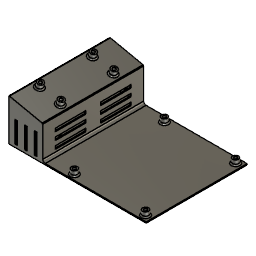
Assembly (Autodesk Fusion 360 archive; units mm, degrees)
design "Chassis"
Autodesk Fusion 360 part; units mm, degrees
sketch "Sketch1" plane through (0, 0, 0) normal (0, 1, 0) x (1, 0, 0)
  line L0 (-55.7763, -66.6431) -> (-54.7763, -66.6431)
  line L1 (-54.7763, -66.6431) -> (0, -55)
  line L2 (0, -55) -> (0, 0)
  line L3 (0, 0) -> (170, 0)
  line L4 (170, 0) -> (170, 2)
  line L5 (170, 2) -> (-55.7763, 2)
  line L6 (-55.7763, 2) -> (-55.7763, -66.6431)
  dimension "d4" = 1
  dimension "d5" = 170
  dimension "d6" = 2
  dimension "d7" = 56
  dimension "d8" = 55
  dimension "d9" = 12
  constraint horizontal L0
  constraint coincident L2.end L3.start
  constraint vertical L2
  constraint perpendicular L2 L3
  constraint perpendicular L3 L4
  constraint perpendicular L4 L5
  constraint perpendicular L0 L6
  measures "d4" distance of L0.start L0.end
  measures "d5" distance of L2.end L3.end
  measures "d6" distance of L3.end L4.end
  measures "d7" distance of L0.end L1.end
  measures "d8" distance of L1.end L2.end
  measures "d9" angle of L1 L3
extrude "Extrude1" add sketch "Sketch1" along normal mid plane 166
fillet "Fillet1" radius 4 1 edges at (0, 0, 0)
chamfer "Chamfer1" distance 1 angle 45 1 edges at (0, 0, 55)
shell "Shell3" thickness 1.8 removed faces 0 bodies 1
sketch "Sketch2" plane through (0, 0, 0) normal (0, 0, 1) x (-1, 0, 0)
  line L0 (-4, -83) -> (-4, 83)
  line L1 (-4, 83) -> (-170, 83)
  line L2 (-170, 83) -> (-170, -83)
  line L3 (-170, -83) -> (-4, -83)
  line L4 (-43, 74) -> (-160, 74) construction
  line L5 (-160, 74) -> (-160, -74) construction
  line L6 (-160, -74) -> (-43, -74) construction
  line L7 (-43, -74) -> (-43, 74) construction
  circle A0 centre (-43, 74) radius 5
  circle A1 centre (-43, -74) radius 5
  circle A2 centre (-160, 74) radius 5
  circle A3 centre (-160, -74) radius 5
  point P0 (-43, 0)
  dimension "d14" = 117
  dimension "d15" = 148
  dimension "d17" = 10
  dimension "d18" = 10
  constraint horizontal L4
  constraint vertical L5
  constraint horizontal L6
  constraint vertical L7
  constraint midpoint L7 P0
  constraint horizontal origin P0
  constraint coincident L4.start L7.end
  constraint coincident L6.end L7.start
  constraint equal A0 A1
  constraint coincident L4.end L5.start
  constraint coincident L5.end L6.start
  constraint equal A0 A2
  constraint equal A0 A3
  measures "d14" distance of L4.start L4.end
  measures "d15" distance of L4.start L6.end
  measures "d17" distance of L2 L5
  measures "d18" diameter of A0
extrude "Extrude2" add sketch "Sketch2" along normal blind 8 contours A0 | A1 | A2 | A3
sketch "Sketch3" plane through (11.1853, 0, 52.6225) normal (0.207912, 0, 0.978148) x (0, 1, 0)
  line L0 (83, 12.4351) -> (83, 67.4351)
  line L1 (83, 67.4351) -> (-83, 67.4351)
  line L2 (-83, 67.4351) -> (-83, 12.4351)
  line L3 (-43.5, 57.4351) -> (43.5, 57.4351) construction
  line L4 (43.5, 57.4351) -> (43.5, 22.4351) construction
  line L5 (43.5, 22.4351) -> (-43.5, 22.4351) construction
  line L6 (-43.5, 22.4351) -> (-43.5, 57.4351) construction
  circle A0 centre (-43.5, 57.4351) radius 5
  circle A1 centre (43.5, 57.4351) radius 5
  circle A2 centre (-43.5, 22.4351) radius 5
  circle A3 centre (43.5, 22.4351) radius 5
  line L7 (-83, 12.4351) -> (83, 12.4351)
  point P0 (0, 22.4351)
  point P1 (0, 10.3528)
  dimension "d21" = 87
  dimension "d22" = 35
  dimension "d23" = 10
  dimension "d24" = 10
  constraint horizontal L3
  constraint vertical L4
  constraint horizontal L5
  constraint vertical L6
  constraint midpoint L5 P0
  constraint vertical P0 P1
  constraint coincident L3.start L6.end
  constraint coincident L3.end L4.start
  constraint coincident L5.end L6.start
  constraint coincident L4.end L5.start
  constraint equal A0 A2
  constraint equal A1 A2
  constraint equal A1 A3
  measures "d21" distance of L3.start L3.end
  measures "d22" distance of L3.start L5.end
  measures "d23" distance of L1 L3
  measures "d24" diameter of A0
extrude "Extrude3" add sketch "Sketch3" along normal blind 8 contours A0 | A1 | A2 | A3
sketch "Sketch5" plane through (12.8486, 0, 60.4477) normal (0.207912, 0, 0.978148) x (0, 1, 0)
  circle A0 centre (-43.5, 57.4351) radius 5
  circle A1 centre (43.5, 57.4351) radius 5
  circle A2 centre (-43.5, 22.4351) radius 5
  circle A3 centre (43.5, 22.4351) radius 5
  point P0 (-43.5, 57.4351)
  point P1 (43.5, 57.4351)
  point P2 (43.5, 22.4351)
  point P3 (-43.5, 22.4351)
  constraint coincident P0 A0.centre
  constraint coincident P1 A1.centre
  constraint coincident P2 A3.centre
  constraint coincident A2.centre P3
hole "Hole1" at (-9.0963, -43.5, 65.1122) at (-43.3315, -43.5, 72.3891) at (-9.0963, 43.5, 65.1122) at (-43.3315, 43.5, 72.3891) direction (-0.207912, 0, -0.978148) diameter 4.5 depth 6 tip angle 180 countersink diameter 5.2 countersink angle 90
sketch "Sketch6" plane through (0, 0, 8) normal (0, 0, 1) x (-1, 0, 0)
  circle A0 centre (-43, 74) radius 5
  circle A1 centre (-43, -74) radius 5
  circle A2 centre (-160, -74) radius 5
  circle A3 centre (-160, 74) radius 5
  point P0 (-43, -74)
  point P1 (-160, -74)
  point P2 (-43, 74)
  point P3 (-160, 74)
  constraint coincident P0 A1.centre
  constraint coincident P1 A2.centre
  constraint coincident P2 A0.centre
  constraint coincident P3 A3.centre
hole "Hole2" at (43, -74, 8) at (43, 74, 8) at (160, 74, 8) at (160, -74, 8) direction (0, 0, -1) diameter 4.5 depth 6 tip angle 180 countersink diameter 5.2 countersink angle 90
fillet "Fillet3" radius 2 4 edges at (47.6616, -75.8081, 0) (47.6616, 72.1919, 0) (164.6616, -75.8081, 0) (164.6616, 72.1919, 0)
fillet "Fillet4" radius 2 4 edges at (-46.7634, 38.8384, 64.9399) (-46.7634, -48.1616, 64.9399) (-12.5282, -48.1616, 57.6629) (-12.5282, 38.8384, 57.6629)
sketch "Sketch8" plane through (-55.7763, 0, 0) normal (-1, 0, 0) x (0, -1, 0)
  line L0 (83, 66.6431) -> (-83, 66.6431)
  line L1 (-83, 66.6431) -> (-83, -2)
  line L2 (-83, -2) -> (83, -2)
  line L3 (83, -2) -> (83, 66.6431)
  line L4 (-62.1541, 13) -> (-12.1541, 13)
  line L5 (-12.1541, 13) -> (-12.1541, 8)
  line L6 (-12.1541, 8) -> (-62.1541, 8)
  line L7 (-62.1541, 8) -> (-62.1541, 13)
  line L8 (12.1541, 13) -> (62.1541, 13)
  line L9 (62.1541, 13) -> (62.1541, 8)
  line L10 (62.1541, 8) -> (12.1541, 8)
  line L11 (12.1541, 8) -> (12.1541, 13)
  line L12 (0, 1.75) -> (0, 22.5)
  dimension "d95" = 50
  dimension "d96" = 5
  dimension "d99" = 10
  constraint horizontal L4
  constraint vertical L5
  constraint horizontal L6
  constraint vertical L7
  constraint horizontal L8
  constraint vertical L9
  constraint horizontal L10
  constraint vertical L11
  constraint equal L4 L8
  constraint equal L5 L11
  constraint symmetric L4 L8 L12
  measures "d95" distance of L4.start L4.end
  measures "d96" distance of L4.start L6.end
  measures "d99" distance of L2 L6
extrude "Extrude5" cut sketch "Sketch8" against normal blind 90 contours L4 L5 L6 L7 | L8 L9 L10 L11
pattern_linear "R-Pattern1" count 3 spacing 12.5 along (0, 0, 1) of "Extrude5"
sketch "Sketch10" plane through (0, -83, 0) normal (0, -1, 0) x (1, 0, 0)
  line L0 (0, 54) -> (-0.9781, 55.2079)
  line L1 (-0.9781, 55.2079) -> (-54.7763, 66.6431)
  line L2 (-54.7763, 66.6431) -> (-55.7763, 66.6431)
  line L3 (-55.7763, 66.6431) -> (-55.7763, -2)
  line L4 (-55.7763, -2) -> (170, -2)
  line L5 (170, -2) -> (170, 0)
  line L6 (170, 0) -> (4, 0)
  arc A0 (0, 4) -> (4, 0) centre (4, 4) ccw
  line L7 (0, 4) -> (0, 54)
  line L8 (-45.7763, 38) -> (-41.7763, 38)
  line L9 (-41.7763, 38) -> (-41.7763, 3)
  line L10 (-41.7763, 3) -> (-45.7763, 3)
  line L11 (-45.7763, 3) -> (-45.7763, 38)
  dimension "d76" = 5
  dimension "d77" = 10
  dimension "d78" = 4
  dimension "d94" = 35
  constraint horizontal L8
  constraint vertical L9
  constraint horizontal L10
  constraint vertical L11
  measures "d76" distance of L4 L10
  measures "d77" distance of L3 L11
  measures "d78" distance of L8.start L8.end
  measures "d94" distance of L8.end L9.end
extrude "Extrude7" cut sketch "Sketch10" against normal blind 170 contours L8 L9 L10 L11
pattern_linear "R-Pattern2" count 3 spacing 16 along (1, 0, 0) of "Extrude7"
sketch "Sketch9" plane through (0, 0, -2) normal (0, 0, -1) x (1, 0, 0)
  line L0 (-55.7763, 83) -> (-55.7763, -83)
  line L1 (-55.7763, -83) -> (170, -83)
  line L2 (170, -83) -> (170, 83)
  line L3 (170, 83) -> (-55.7763, 83)
  circle A0 centre (-27.8881, -30) radius 2
  circle A1 centre (-27.8881, 30) radius 2
  line L4 (1.75, 0) -> (22.5, 0)
  line L5 (-27.8881, 83) -> (-27.8881, -83) construction
  line L6 (-55.7763, -83) -> (-55.7763, 83)
  line L7 (0, 0) -> (-55.7763, 0) construction
  circle A2 centre (-27.8881, -30) radius 1
  circle A3 centre (-27.8881, 30) radius 1
  dimension "d70" = 4
  dimension "d71" = 60
  dimension "d93" = 2
  constraint equal A0 A1
  constraint symmetric A0 A1 L4
  constraint coincident L3 L5.start
  constraint coincident L1 L5.end
  constraint perpendicular L1 L5
  constraint coincident L7.start origin
  constraint midpoint L6 L7.end
  constraint midpoint L5 L7
  constraint coincident A0.centre L5
  constraint concentric A0 A2
  constraint concentric A1 A3
  constraint equal A2 A3
  measures "d70" diameter of A0
  measures "d71" distance of A0.centre A1.centre
  measures "d93" diameter of A2
extrude "Extrude6" add sketch "Sketch9" along normal up to surface contours A0 | A1 end surface through (-54.7763, 0, 66.6431) normal (0.207912, 0, 0.978148) offset 0
fillet "Fillet5" radius 2 4 edges at (-29.7528, -29.2768, -0.2) (-29.7528, 30.7232, -0.2) (-29.8881, 30, 59.5127) (-29.8881, -30, 59.5127)

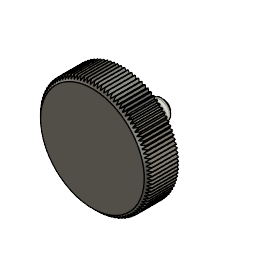
design "Knurled Thumb Screw DIN 653 - M1 x 2 Steel 4.6 Plain"
description: Knurled Thumb Screw DIN 653 - M1 x 2
part number: DIN 653 - M1 x 2 Steel 4.6 Plain
Autodesk Fusion 360 part; units mm, degrees
sketch "Sketch1" plane through (0, 0, 0) normal (0, 1, 0) x (1, 0, 0)
  line L0 (0, 2) -> (0, -1.5)
  line L1 (0, -1.5) -> (-2.55, -1.5)
  line L2 (-2.75, -1.3) -> (-2.75, 0)
  line L3 (-2.75, 0) -> (-1, 0)
  line L4 (-0.5, 0.5) -> (-0.5, 2)
  line L5 (-0.5, 2) -> (0, 2)
  arc A0 (-1, 0) -> (-0.5, 0.5) centre (-1, 0.5) ccw
  line L6 (-2.55, -1.5) -> (-2.75, -1.3)
  dimension "d222" = 1
  dimension "d223" = 2
  dimension "d250" = 0.5
  dimension "d257" = 135
  dimension "d258" = 5.5
  dimension "d259" = 1.5
  dimension "d260" = 0.2
  constraint vertical L0
  constraint coincident L0.end L1
  constraint coincident L0 L1.start
  constraint coincident origin L0
  constraint coincident origin L3
  constraint coincident L0 L5.end
  constraint perpendicular L0 L5
  constraint coincident L0.start L5
  constraint tangent L3 A0
  constraint tangent L4 A0
  constraint horizontal L1
  measures "d223" distance of origin L5
  measures "d250" distance of L4 A0.centre
  measures "d257" angle of L1 L6
  measures "d259" distance of L1 L3
  measures "d260" distance of L1 L2.start
revolve "Revolve1" add sketch "Sketch1" angle 360 about axis through (0, 0, -2) along (0, 0, 1)
sketch "Sketch22" plane through (0, 0, 1.5) normal (0, 0, 1) x (1, 0, 0)
  line L0 (-0.0787, 2.7489) -> (0, 2.6125)
  line L1 (0, 2.6125) -> (0.0787, 2.7489)
  line L2 (0, 0) -> (0, 2.75) construction
  arc A0 (0.0787, 2.7489) -> (-0.0787, 2.7489) centre (0, 0) ccw
  line L3 (0, 0) -> (-2.75, 0) construction
  circle A1 centre (0, 0) radius 2.75
  dimension "d169" = 60
  dimension "d186" = 150
  dimension "d252" = 2.6125
  constraint coincident L0.end L2
  constraint coincident L2.start A0.centre
  constraint coincident A0.centre L2
  constraint vertical L2
  constraint coincident L2.end A0
  constraint coincident L3.end A1
  constraint perpendicular L2 L3
  constraint coincident L2.end A1
  measures "d169" angle of L0 L1
  measures "d186" angle of L0 L2
  measures "d252" distance of L0.end L3
extrude "Extrude11" cut sketch "Sketch22" against normal blind 1.5 contours L0 L1 A0 A1
pattern_circular "C-Pattern4" count 100 over 360 about axis through (0, 0, 1.75) along (0, 0, 1) of "Extrude11"
thread "Thread5" "ISO Metric profile 1.0 M1x0.25 M1x0.25 6g" major diameter 0.9485 minor diameter 0.662 pitch 0.25 angle 60 resizes the face on face at (-0.4975, 0.0498, -1.5)
sketch "Sketch23" plane through (0, 0, 0) normal (0, 1, 0) x (1, 0, 0)
  line L0 (0, 2) -> (0, -1.5)
  line L1 (-0.51, 1.8466) -> (-0.51, 2)
  line L2 (-0.51, 2) -> (0, 2)
  line L3 (-0.51, 1.8466) -> (-0.3466, 2)
  dimension "d254" = 0.51
  dimension "d255" = 0.3466
  dimension "d256" = 0.1534
  constraint coincident L0.start L2.end
  constraint perpendicular L1 L2
  constraint perpendicular L0 L2
  constraint coincident L2 L3.end
  measures "d254" distance of L1 L0.start
  measures "d255" distance of L0 L3.end
  measures "d256" distance of L1.start L2
revolve "Revolve5" cut sketch "Sketch23" angle 360 about axis through (0, 0, 1.75) along (0, 0, 1)
equation "adsk_headdia = 5.50 mm"
equation "adsk_nomdia = 1.00 mm"
equation "adsk_nomlen = 2.00 mm"
equation "adsk_chamheig = 0.20 mm"
equation "d173 = -adsk_headh"
equation "adsk_headh = 1.50 mm"
equation "d222 = adsk_nomdia"
equation "d223 = adsk_nomlen"
equation "adsk_midfillet = 0.50 mm"
equation "adsk_startlen = 0.153363 mm"
equation "adsk_endpointdia = 0.693275 mm"
equation "d250 = adsk_midfillet"
equation "d252 = 0.95 * adsk_headdia / 2"
equation "d254 = adsk_nomdia * 0.51"
equation "d255 = adsk_endpointdia / 2"
equation "d256 = adsk_startlen"
equation "d257 = 180 deg - 45 deg"
equation "d258 = adsk_headdia"
equation "d259 = adsk_headh"
equation "d260 = adsk_chamheig"
